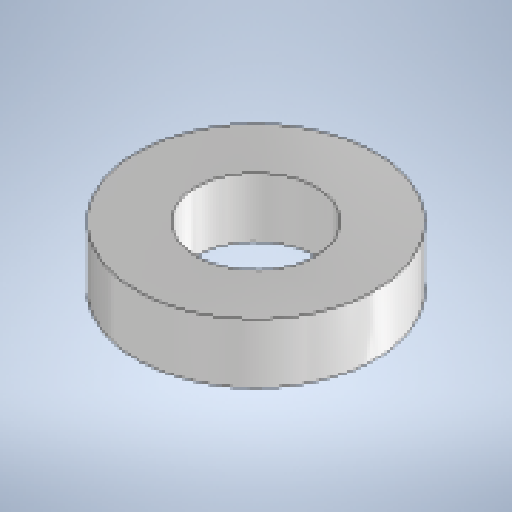
# Autodesk Inventor part: Gear
Saved by Autodesk Inventor 2023.2 (Build 272271000, 271)
## iProperties
Created: 2024-02-03
Part Number: Gear
Material: Nylon 6/6
Document SubType Name: Modeling
Designer: Nathan Cai
Density: 1.13 g/cm^3
Appearance: Nylon 6
Author: Nathan Cai
Autodesk Inventor part; units mm, degrees
ref_plane "YZ Plane" through (0, 0, 0) normal (1, 0, 0) x (0, 1, 0)
ref_plane "XZ Plane" through (0, 0, 0) normal (0, 1, 0) x (-1, 0, 0)
ref_plane "XY Plane" through (0, 0, 0) normal (0, 0, 1) x (1, 0, 0)
sketch "Sketch1" plane through (0, 0, 0) normal (0, 1, 0) x (-1, 0, 0)
  circle A0 centre (0, 0) radius 6.35
  circle A1 centre (0, 0) radius 12.7
  circle A2 centre (0, 0) radius 9.525 construction
  line L0 (0, 9.525) -> (0, 0) construction
  circle A3 centre (0, 9.525) radius 1.7526
  circle A4 centre (-8.2489, 4.7625) radius 1.7526
  circle A5 centre (-8.2489, -4.7625) radius 1.7526
  circle A6 centre (0, -9.525) radius 1.7526
  circle A7 centre (8.2489, -4.7625) radius 1.7526
  circle A8 centre (8.2489, 4.7625) radius 1.7526
  dimension "d4" = 19.05
  dimension "d0" = 12.7
  dimension "d1" = 25.4
  dimension "d5" = 3.5052
  dimension "d8" = 360
  constraints: 8 centre point, 4 coincident, 2 end point, 1 vertical, 1 vertical alignment, 15 other
  measures "d0" diameter of A0
  measures "d1" diameter of A1
  measures "d5" diameter of A3
extrude "Extrusion1" add sketch "Sketch1" along normal blind 6.35
body "Solid1"
